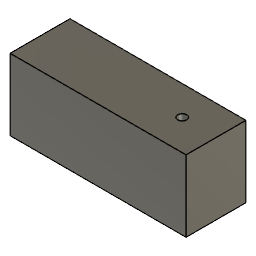
モーター (Autodesk Fusion 360 design; units mm, degrees)
Autodesk Fusion 360 part; units mm, degrees
sketch "スケッチ1" plane through (0, 0, 0) normal (0, 0, 1) x (1, 0, 0)
  line L0 (0, 0) -> (69, 0)
  line L1 (69, 0) -> (69, 23.5)
  line L2 (69, 23.5) -> (0, 23.5)
  line L3 (0, 23.5) -> (0, 0)
  circle A0 centre (55.5, 12) radius 1.75
  dimension "d1" = 12
  dimension "d2" = 3.5
  dimension "d3" = 23.5
  dimension "d4" = 69
  dimension "d5" = 13.5
  constraint horizontal L0
  constraint vertical L1
  constraint horizontal L2
  constraint vertical L3
  constraint coincident L0.start L3.end
  measures "d1" distance of L0 A0.centre
  measures "d2" diameter of A0
  measures "d3" distance of L0.end L1.end
  measures "d4" distance of L1.end L2.end
  measures "d5" distance of L1 A0.centre
extrude "押し出し1" add sketch "スケッチ1" along normal blind 28
